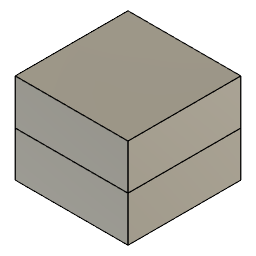
box (Autodesk Fusion 360 design; units mm, degrees)
part number: 2025-09-21-15-33-46-252
part number: 2025-09-21-15-36-33-395
part number: 2025-09-21-15-40-00-997
Autodesk Fusion 360 part; units mm, degrees
sketch "Box Width" plane through (0, 0, 0) normal (0, 0, 1) x (1, 0, 0) in component "Box Bottom"
  line L0 (0, 0) -> (50, 0)
  line L1 (50, 0) -> (50, 50)
  line L2 (50, 50) -> (0, 50)
  line L3 (0, 50) -> (0, 0)
  dimension "d3" = 50
  dimension "d4" = 50
  constraint horizontal L0
  constraint vertical L1
  constraint horizontal L2
  constraint vertical L3
  constraint coincident L0.start L3.end
  measures "d3" distance of L0.start L0.end
  measures "d4" distance of L0.start L2.end
extrude "Extrude1" add sketch "Box Width" along normal blind 20 makes body 1 in component "Box Bottom"
shell "Shell1" thickness 2 removed faces 1 at (16.6667, 33.3333, 20) on bodies 1 in component "Box Bottom"
sketch "Box Width (2)" plane through (0, 0, 0) normal (0, 0, 1) x (1, 0, 0) in component "Box Top"
  line L0 (0, 0) -> (50, 0)
  line L1 (50, 0) -> (50, 50)
  line L2 (50, 50) -> (0, 50)
  line L3 (0, 50) -> (0, 0)
  dimension "d3_1" = 50
  dimension "d4_1" = 50
  constraint horizontal L0
  constraint vertical L1
  constraint horizontal L2
  constraint vertical L3
  constraint coincident L0.start L3.end
  measures "d3_1" distance of L0.start L0.end
  measures "d4_1" distance of L0.start L2.end
extrude "Extrude1'" add sketch "Box Width (2)" along normal blind 20 separate body makes body 2 in component "Box Top"
shell "Shell1'" thickness 2 removed faces 1 at (16.6667, 33.3333, 20) on bodies 2 in component "Box Top"
component "Box Bottom" placed x (1, 0, 0) y (0, 1, 0) z (0, 0, 1) at (0, 0, 0)
component "Box Top" placed x (0, 1, 0) y (1, 0, 0) z (0, 0, -1) at (0, 0, 40)
equation "BoxWidth = 50 mm"
equation "BoxHeight = 40 mm"
equation "d3 = BoxWidth"
equation "d4 = BoxWidth"
equation "d5 = BoxHeight / 2"
equation "WallThickness = 2 mm"
equation "d3_1 = BoxWidth"
equation "d4_1 = BoxWidth"
equation "d5_1 = BoxHeight / 2"
equation "WallThickness_1 = 2 mm"
